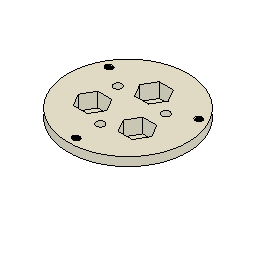
bottom platform (Autodesk Fusion 360 design; units mm, degrees)
Autodesk Fusion 360 part; units mm, degrees
sketch "Sketch6" plane through (0, 0, 0) normal (0, 1, 0) x (1, 0, 0)
  circle A0 centre (0, 0) radius 32.5
  dimension "d28" = 65
  constraint coincident A0.centre origin
  measures "d28" diameter of A0
extrude "Extrude5" add sketch "Sketch6" along normal blind 10 makes body 1
sketch "Sketch7" plane through (0, 0, 0) normal (0, -1, 0) x (1, 0, 0)
  circle A0 centre (0, 0) radius 32.5
  circle A1 centre (0, 0) radius 6
  dimension "d31" = 12
  constraint coincident A0.centre A1.centre
  measures "d31" diameter of A1
extrude "Extrude6" add sketch "Sketch7" along normal blind 10 contours A1 bodies 1
fillet "Fillet5" radius 3 1 edges at (-5.594, 0, 2.1697) on bodies 1
sketch "Sketch8" plane through (0, -10, 0) normal (0, -1, 0) x (1, 0, 0)
  circle A0 centre (0, 0) radius 6
  circle A1 centre (0, 0) radius 3.175
  dimension "d36" = 6.35
  constraint coincident A0.centre A1.centre
  measures "d36" diameter of A1
extrude "Extrude7" cut sketch "Sketch8" against normal blind 15 contours A1 bodies 1
thread "Thread2" "ANSI Unified Screw Threads 0.25 1/4-20 UNC 3B" major diameter 6.35 minor diameter 5.1156 pitch 1.27 angle 60 modelled right hand crest width 0.3725 on face at (3.1592, 0, -0.3161) crest through (2.5578, -9.6825, 0) on bodies 1
sketch "Sketch9" plane through (0, 10, 0) normal (0, 1, 0) x (-1, 0, 0)
  circle A0 centre (0, 0) radius 32.5
  circle A1 centre (0, 0) radius 23
  circle A2 centre (0, 0) radius 15 construction
  line L0 (4.1095, -22.0963) -> (8.2024, -14.9927)
  line L1 (8.2024, -14.9927) -> (4.0969, -7.8964)
  line L2 (4.0969, -7.8964) -> (-4.1015, -7.9037)
  line L3 (-4.1015, -7.9037) -> (-8.1944, -15.0073)
  line L4 (-8.1944, -15.0073) -> (-4.0889, -22.1036)
  line L5 (-4.0889, -22.1036) -> (4.1095, -22.0963)
  line L6 (21.1868, 7.5108) -> (17.0812, 14.6071)
  line L7 (17.0812, 14.6071) -> (8.8829, 14.5998)
  line L8 (8.8829, 14.5998) -> (4.79, 7.4962)
  line L9 (4.79, 7.4962) -> (8.8955, 0.3998)
  line L10 (8.8955, 0.3998) -> (17.0939, 0.4071)
  line L11 (17.0939, 0.4071) -> (21.1868, 7.5108)
  line L12 (-17.0979, 14.5929) -> (-21.1907, 7.4892)
  line L13 (-21.1907, 7.4892) -> (-17.0852, 0.3929)
  line L14 (-17.0852, 0.3929) -> (-8.8869, 0.4002)
  line L15 (-8.8869, 0.4002) -> (-4.794, 7.5038)
  line L16 (-4.794, 7.5038) -> (-8.8995, 14.6002)
  line L17 (-8.8995, 14.6002) -> (-17.0979, 14.5929)
  point P0 (0.004, -15)
  dimension "d39" = 46
  dimension "d40" = 30
  dimension "d41" = 14.2
  dimension "d43" = 360
  constraint coincident A0.centre A1.centre
  constraint coincident A2 P0
  measures "d39" diameter of A1
  measures "d40" diameter of A2
  measures "d41" distance of L2 L5
extrude "Extrude8" cut sketch "Sketch9" against normal blind 8.382 contours L0 L1 L2 L3 L4 L5 | L6 L7 L8 L9 L10 L11 | L12 L13 L14 L15 L16 L17 bodies 1
sketch "Sketch11" plane through (0, 0, 0) normal (0, -1, 0) x (1, 0, 0)
  circle A0 centre (0, 0) radius 32.5
  circle A1 centre (0, 0) radius 9
  circle A2 centre (0, 0) radius 27.5
  dimension "d65" = 55
  constraint concentric A0 A2
  measures "d65" diameter of A2
extrude "Extrude9" cut sketch "Sketch11" against normal blind 5 contours A0 bodies 1
sketch "Sketch12" plane through (0, 5, 0) normal (0, -1, 0) x (1, 0, 0)
  circle A0 centre (0, 0) radius 27.5
  circle A1 centre (0, 0) radius 32.5
  circle A2 centre (25.9808, -15) radius 2
  circle A3 centre (0, 30) radius 2
  line L0 (-28.1458, 16.25) -> (0, 0) construction
  line L1 (0, 0) -> (28.1458, -16.25) construction
  line L2 (0, 0) -> (0, 32.5) construction
  line L3 (23.8157, -13.75) -> (28.1458, -16.25) construction
  line L4 (0, 27.5) -> (0, 32.5) construction
  circle A4 centre (-25.9808, -15) radius 2
  dimension "d68" = 4
  dimension "d69" = 4
  dimension "d78" = 60
  constraint coincident A1 L0.start
  constraint coincident A0.centre A1.centre
  constraint coincident A1 L1.end
  constraint parallel L0 L1
  constraint coincident A1 L2.end
  constraint vertical L2
  constraint coincident A0 L3.start
  constraint coincident L1 L3.start
  constraint midpoint A2.centre L3
  constraint coincident L2 L4.start
  constraint coincident A0 L4.start
  constraint midpoint A3.centre L4
  constraint symmetric A2 L2 A4
  measures "d68" diameter of A2
  measures "d69" diameter of A3
  measures "d78" angle of L0 L2
extrude "Extrude10" cut sketch "Sketch12" against normal blind 5 contours A2 | A3 | A4 bodies 1
thread "Thread4" "ANSI Unified Screw Threads 0.164(#8) 8-32 UNC 3B" major diameter 4.1656 minor diameter 3.4163 pitch 0.7937 angle 60 modelled right hand crest width 0.2414 on face at (27.9783, 8.3333, -15.0997) crest through (27.6889, 5.1984, -15) on face at (-23.9832, 8.3333, -15.0997) crest through (-24.2726, 5.1984, -15) on face at (1.9975, 8.3333, 29.9003) crest through (1.7082, 5.1984, 30) on bodies 1
sketch "Sketch13" plane through (0, 0, 0) normal (0, -1, 0) x (1, 0, 0)
  circle A0 centre (0, 0) radius 27.5
  circle A1 centre (0, 0) radius 9
  line L0 (-8.2024, -14.9927) -> (-4.1095, -22.0963)
  line L1 (-4.1095, -22.0963) -> (4.0889, -22.1036)
  line L2 (4.0889, -22.1036) -> (8.1944, -15.0073)
  line L3 (8.1944, -15.0073) -> (4.1015, -7.9037)
  line L4 (4.1015, -7.9037) -> (-4.0969, -7.8964)
  line L5 (-4.0969, -7.8964) -> (-8.2024, -14.9927)
  line L6 (-17.0812, 14.6071) -> (-21.1868, 7.5108)
  line L7 (-21.1868, 7.5108) -> (-17.0939, 0.4071)
  line L8 (-17.0939, 0.4071) -> (-8.8955, 0.3998)
  line L9 (-8.8955, 0.3998) -> (-4.79, 7.4962)
  line L10 (-4.79, 7.4962) -> (-8.8829, 14.5998)
  line L11 (-8.8829, 14.5998) -> (-17.0812, 14.6071)
  line L12 (21.1907, 7.4892) -> (17.0979, 14.5929)
  line L13 (17.0979, 14.5929) -> (8.8995, 14.6002)
  line L14 (8.8995, 14.6002) -> (4.794, 7.5038)
  line L15 (4.794, 7.5038) -> (8.8869, 0.4002)
  line L16 (8.8869, 0.4002) -> (17.0852, 0.3929)
  line L17 (17.0852, 0.3929) -> (21.1907, 7.4892)
  circle A2 centre (0, 0) radius 32.5
  line L18 (0, 32.5) -> (0, -32.5) construction
  line L19 (-17.1424, 21.5032) -> (0, 9.5)
  line L20 (17.1424, 21.5032) -> (0, 9.5)
  line L21 (-10.0511, -25.5974) -> (-8.2272, -4.75)
  line L22 (-27.1935, 4.0941) -> (-8.2272, -4.75)
  line L23 (27.1935, 4.0941) -> (8.2272, -4.75)
  line L24 (10.0511, -25.5974) -> (8.2272, -4.75)
  spline S0 degree 3 poles (23.9261, -15.3413) (23.9965, -15.5962) (24.115, -15.8353) (24.432, -16.2447) (24.624, -16.4135) (25.0536, -16.6608) (25.2849, -16.7405) (25.6924, -16.7949) (25.862, -16.7938) (26.1902, -16.7441) (26.3473, -16.6973) (26.4954, -16.6288) knots 0 0 0 0 0.079347 0.079347 0.155456 0.155456 0.228326 0.228326 0.279114 0.279114 0.328226 0.328226 0.328226 0.328226
  arc A3 (26.4954, -16.6288) -> (27.3444, -13.9712) centre (25.9808, -15) ccw
  spline S1 degree 3 poles (27.3444, -13.9712) (27.2323, -13.7751) (27.0822, -13.6032) (26.7172, -13.3183) (26.5032, -13.2113) (26.0362, -13.0802) (25.7865, -13.0615) (25.3537, -13.1118) (25.1715, -13.1602) (24.8207, -13.3083) (24.6544, -13.4087) (24.5045, -13.5307) knots 0 0 0 0 0.06777 0.06777 0.138771 0.138771 0.213001 0.213001 0.26909 0.26909 0.326867 0.326867 0.326867 0.326867
  spline S2 degree 3 poles (-2.0546, 29.6587) (-1.9843, 29.4038) (-1.8658, 29.1647) (-1.5488, 28.7553) (-1.3567, 28.5865) (-0.9271, 28.3392) (-0.6958, 28.2595) (-0.2884, 28.2051) (-0.1188, 28.2062) (0.2094, 28.2559) (0.3666, 28.3027) (0.5146, 28.3712) knots 0 0 0 0 0.079347 0.079347 0.155456 0.155456 0.228326 0.228326 0.279114 0.279114 0.328226 0.328226 0.328226 0.328226
  arc A4 (0.5146, 28.3712) -> (1.3636, 31.0288) centre (0, 30) ccw
  spline S3 degree 3 poles (1.3636, 31.0288) (1.2516, 31.2249) (1.1015, 31.3968) (0.7364, 31.6817) (0.5225, 31.7887) (0.0554, 31.9198) (-0.1943, 31.9385) (-0.627, 31.8882) (-0.8092, 31.8398) (-1.1601, 31.6917) (-1.3263, 31.5913) (-1.4763, 31.4693) knots 0 0 0 0 0.06777 0.06777 0.138771 0.138771 0.213001 0.213001 0.26909 0.26909 0.326867 0.326867 0.326867 0.326867
  spline S4 degree 3 poles (-28.0354, -15.3413) (-27.965, -15.5962) (-27.8465, -15.8353) (-27.5296, -16.2447) (-27.3375, -16.4135) (-26.9079, -16.6608) (-26.6766, -16.7405) (-26.2692, -16.7949) (-26.0995, -16.7938) (-25.7713, -16.7441) (-25.6142, -16.6973) (-25.4661, -16.6288) knots 0 0 0 0 0.079347 0.079347 0.155456 0.155456 0.228326 0.228326 0.279114 0.279114 0.328226 0.328226 0.328226 0.328226
  arc A5 (-25.4661, -16.6288) -> (-24.6172, -13.9712) centre (-25.9808, -15) ccw
  spline S5 degree 3 poles (-24.6172, -13.9712) (-24.7292, -13.7751) (-24.8793, -13.6032) (-25.2443, -13.3183) (-25.4583, -13.2113) (-25.9253, -13.0802) (-26.175, -13.0615) (-26.6078, -13.1118) (-26.79, -13.1602) (-27.1408, -13.3083) (-27.3071, -13.4087) (-27.457, -13.5307) knots 0 0 0 0 0.06777 0.06777 0.138771 0.138771 0.213001 0.213001 0.26909 0.26909 0.326867 0.326867 0.326867 0.326867
  arc A6 (-27.457, -13.5307) -> (-28.0354, -15.3413) centre (-25.9808, -15) ccw
  arc A7 (-1.4763, 31.4693) -> (-2.0546, 29.6587) centre (0, 30) ccw
  arc A8 (24.5045, -13.5307) -> (23.9261, -15.3413) centre (25.9808, -15) ccw
  dimension "d72" = 55
  dimension "d73" = 23
  dimension "d75" = 360
  constraint coincident A2 L18.start
  constraint coincident A2 L18.end
  constraint vertical L18
  constraint coincident A0 L19.start
  constraint coincident L18 L19.end
  constraint symmetric L18 L19.start L20.start
  constraint symmetric L18 L19.end L20.end
  measures "d72" angle of L18 L19
  measures "d73" distance of L18.start L19.end
extrude "Extrude11" cut sketch "Sketch13" against normal blind 5 contours A0 L23 L24 | A0 L19 L20 | A0 L21 L22 bodies 1
sketch "Sketch10" plane through (0, 1.618, 0) normal (0, 1, 0) x (-1, 0, 0)
  line L0 (-8.8995, 14.6002) -> (-17.0979, 14.5929)
  line L1 (-17.0979, 14.5929) -> (-21.1907, 7.4892)
  line L2 (-21.1907, 7.4892) -> (-17.0852, 0.3929)
  line L3 (-17.0852, 0.3929) -> (-8.8869, 0.4002)
  line L4 (-8.8869, 0.4002) -> (-4.794, 7.5038)
  line L5 (-4.794, 7.5038) -> (-8.8995, 14.6002)
  line L6 (-4.0889, -22.1036) -> (4.1095, -22.0963)
  line L7 (4.1095, -22.0963) -> (8.2024, -14.9927)
  line L8 (8.2024, -14.9927) -> (4.0969, -7.8964)
  line L9 (4.0969, -7.8964) -> (-4.1015, -7.9037)
  line L10 (-4.1015, -7.9037) -> (-8.1944, -15.0073)
  line L11 (-8.1944, -15.0073) -> (-4.0889, -22.1036)
  line L12 (17.0939, 0.4071) -> (21.1868, 7.5108)
  line L13 (21.1868, 7.5108) -> (17.0812, 14.6071)
  line L14 (17.0812, 14.6071) -> (8.8829, 14.5998)
  line L15 (8.8829, 14.5998) -> (4.79, 7.4962)
  line L16 (4.79, 7.4962) -> (8.8955, 0.3998)
  line L17 (8.8955, 0.3998) -> (17.0939, 0.4071)
  line L18 (17.0939, 0.4071) -> (21.1868, 7.5108)
  line L19 (21.1868, 7.5108) -> (17.0812, 14.6071)
  line L20 (17.0812, 14.6071) -> (8.8829, 14.5998)
  line L21 (8.8829, 14.5998) -> (4.79, 7.4962)
  line L22 (4.79, 7.4962) -> (8.8955, 0.3998)
  line L23 (8.8955, 0.3998) -> (17.0939, 0.4071)
  line L24 (4.1095, -22.0963) -> (8.2024, -14.9927)
  line L25 (8.2024, -14.9927) -> (4.0969, -7.8964)
  line L26 (4.0969, -7.8964) -> (-4.1015, -7.9037)
  line L27 (-4.1015, -7.9037) -> (-8.1944, -15.0073)
  line L28 (-8.1944, -15.0073) -> (-4.0889, -22.1036)
  line L29 (-4.0889, -22.1036) -> (4.1095, -22.0963)
  line L30 (-8.8869, 0.4002) -> (-4.794, 7.5038)
  line L31 (-4.794, 7.5038) -> (-8.8995, 14.6002)
  line L32 (-8.8995, 14.6002) -> (-17.0979, 14.5929)
  line L33 (-17.0979, 14.5929) -> (-21.1907, 7.4892)
  line L34 (-21.1907, 7.4892) -> (-17.0852, 0.3929)
  line L35 (-17.0852, 0.3929) -> (-8.8869, 0.4002)
  circle A0 centre (12.9884, 7.5035) radius 3.5
  circle A1 centre (0.004, -15) radius 3.5
  circle A2 centre (-12.9924, 7.4965) radius 3.5
  point P0 (12.9884, 7.5035)
  point P1 (0.004, -15)
  point P2 (-12.9924, 7.4965)
  dimension "d50" = 7
  dimension "d51" = 7
  dimension "d52" = 7
  constraint coincident L16.end L17.start
  constraint coincident L12.start L17.end
  constraint coincident L6.start L11.end
  constraint coincident L6.end L7.start
  constraint coincident L3.end L4.start
  constraint coincident L2.end L3.start
  constraint coincident P0 A0.centre
  constraint coincident P1 A1.centre
  constraint coincident P2 A2.centre
  measures "d50" diameter of A0
  measures "d51" diameter of A1
  measures "d52" diameter of A2
fillet "Fillet7" radius 2 9 edges at (-17.1424, 2.5, 21.5032) (-27.1935, 2.5, 4.0941) (0, 2.5, 9.5) (17.1424, 2.5, 21.5032) (27.1935, 2.5, 4.0941) (8.2272, 2.5, -4.75) (10.0511, 2.5, -25.5974) (-10.0511, 2.5, -25.5974) (-8.2272, 2.5, -4.75) on bodies 1
sketch "Sketch14" plane through (0, 10, 0) normal (0, 1, 0) x (-1, 0, 0)
  line L0 (8.2024, -14.9927) -> (4.1095, -22.0963)
  line L1 (4.1095, -22.0963) -> (-4.0889, -22.1036)
  line L2 (-4.0889, -22.1036) -> (-8.1944, -15.0073)
  line L3 (-8.1944, -15.0073) -> (-4.1015, -7.9037)
  line L4 (-4.1015, -7.9037) -> (4.0969, -7.8964)
  line L5 (4.0969, -7.8964) -> (8.2024, -14.9927)
  line L6 (17.0812, 14.6071) -> (21.1868, 7.5108)
  line L7 (21.1868, 7.5108) -> (17.0939, 0.4071)
  line L8 (17.0939, 0.4071) -> (8.8955, 0.3998)
  line L9 (8.8955, 0.3998) -> (4.79, 7.4962)
  line L10 (4.79, 7.4962) -> (8.8829, 14.5998)
  line L11 (8.8829, 14.5998) -> (17.0812, 14.6071)
  line L12 (-21.1907, 7.4892) -> (-17.0979, 14.5929)
  line L13 (-17.0979, 14.5929) -> (-8.8995, 14.6002)
  line L14 (-8.8995, 14.6002) -> (-4.794, 7.5038)
  line L15 (-4.794, 7.5038) -> (-8.8869, 0.4002)
  line L16 (-8.8869, 0.4002) -> (-17.0852, 0.3929)
  line L17 (-17.0852, 0.3929) -> (-21.1907, 7.4892)
  circle A0 centre (0, 0) radius 32.5
  circle A1 centre (0, 0) radius 25
  circle A2 centre (0.004, -15) radius 3.5
  circle A3 centre (12.9884, 7.5035) radius 3.5
  circle A4 centre (-12.9924, 7.4965) radius 3.5
  circle A5 centre (0.004, -15) radius 4.9784
  circle A6 centre (-12.9924, 7.4965) radius 4.9784
  circle A7 centre (12.9884, 7.5035) radius 4.9784
  line L18 (0, 0) -> (-0.0223, 25) construction
  line L19 (0, 0) -> (21.6618, -12.4807) construction
  line L20 (0, 0) -> (-21.6395, -12.5193) construction
  circle A8 centre (13.8635, -7.9877) radius 2.3
  circle A9 centre (-0.0142, 16) radius 2.3
  circle A10 centre (-13.8493, -8.0123) radius 2.3
  spline S0 degree 3 poles (-23.9261, -15.3413) (-23.9965, -15.5962) (-24.115, -15.8353) (-24.432, -16.2447) (-24.624, -16.4135) (-25.0536, -16.6608) (-25.2849, -16.7405) (-25.6924, -16.7949) (-25.862, -16.7938) (-26.1902, -16.7441) (-26.3473, -16.6973) (-26.4954, -16.6288) knots 0 0 0 0 0.079347 0.079347 0.155456 0.155456 0.228326 0.228326 0.279114 0.279114 0.328226 0.328226 0.328226 0.328226
  arc A11 (-27.3444, -13.9712) -> (-26.4954, -16.6288) centre (-25.9808, -15) ccw
  spline S1 degree 3 poles (-27.3444, -13.9712) (-27.2323, -13.7751) (-27.0822, -13.6032) (-26.7172, -13.3183) (-26.5032, -13.2113) (-26.0362, -13.0802) (-25.7865, -13.0615) (-25.3537, -13.1118) (-25.1715, -13.1602) (-24.8207, -13.3083) (-24.6544, -13.4087) (-24.5045, -13.5307) knots 0 0 0 0 0.06777 0.06777 0.138771 0.138771 0.213001 0.213001 0.26909 0.26909 0.326867 0.326867 0.326867 0.326867
  spline S2 degree 3 poles (2.0546, 29.6587) (1.9843, 29.4038) (1.8658, 29.1647) (1.5488, 28.7553) (1.3567, 28.5865) (0.9271, 28.3392) (0.6958, 28.2595) (0.2884, 28.2051) (0.1188, 28.2062) (-0.2094, 28.2559) (-0.3666, 28.3027) (-0.5146, 28.3712) knots 0 0 0 0 0.079347 0.079347 0.155456 0.155456 0.228326 0.228326 0.279114 0.279114 0.328226 0.328226 0.328226 0.328226
  arc A12 (-1.3636, 31.0288) -> (-0.5146, 28.3712) centre (0, 30) ccw
  spline S3 degree 3 poles (-1.3636, 31.0288) (-1.2516, 31.2249) (-1.1015, 31.3968) (-0.7364, 31.6817) (-0.5225, 31.7887) (-0.0554, 31.9198) (0.1943, 31.9385) (0.627, 31.8882) (0.8092, 31.8398) (1.1601, 31.6917) (1.3263, 31.5913) (1.4763, 31.4693) knots 0 0 0 0 0.06777 0.06777 0.138771 0.138771 0.213001 0.213001 0.26909 0.26909 0.326867 0.326867 0.326867 0.326867
  spline S4 degree 3 poles (28.0354, -15.3413) (27.965, -15.5962) (27.8465, -15.8353) (27.5296, -16.2447) (27.3375, -16.4135) (26.9079, -16.6608) (26.6766, -16.7405) (26.2692, -16.7949) (26.0995, -16.7938) (25.7713, -16.7441) (25.6142, -16.6973) (25.4661, -16.6288) knots 0 0 0 0 0.079347 0.079347 0.155456 0.155456 0.228326 0.228326 0.279114 0.279114 0.328226 0.328226 0.328226 0.328226
  arc A13 (24.6172, -13.9712) -> (25.4661, -16.6288) centre (25.9808, -15) ccw
  spline S5 degree 3 poles (24.6172, -13.9712) (24.7292, -13.7751) (24.8793, -13.6032) (25.2443, -13.3183) (25.4583, -13.2113) (25.9253, -13.0802) (26.175, -13.0615) (26.6078, -13.1118) (26.79, -13.1602) (27.1408, -13.3083) (27.3071, -13.4087) (27.457, -13.5307) knots 0 0 0 0 0.06777 0.06777 0.138771 0.138771 0.213001 0.213001 0.26909 0.26909 0.326867 0.326867 0.326867 0.326867
  arc A14 (28.0354, -15.3413) -> (27.457, -13.5307) centre (25.9808, -15) ccw
  arc A15 (2.0546, 29.6587) -> (1.4763, 31.4693) centre (0, 30) ccw
  arc A16 (-23.9261, -15.3413) -> (-24.5045, -13.5307) centre (-25.9808, -15) ccw
  dimension "d81" = 50
  dimension "d82" = 9.9568
  dimension "d83" = 9.9568
  dimension "d84" = 9.9568
  dimension "d86" = 120
  dimension "d87" = 120
  dimension "d88" = 4.6
  dimension "d89" = 9
  dimension "d91" = 360
  constraint coincident A0.centre A1.centre
  constraint concentric A2 A5
  constraint concentric A4 A6
  constraint concentric A3 A7
  constraint coincident A1 L18.end
  constraint perpendicular L16 L18
  constraint coincident A1 L20.end
  constraint coincident L19 A8.centre
  measures "d81" diameter of A1
  measures "d82" diameter of A5
  measures "d83" diameter of A6
  measures "d84" diameter of A7
  measures "d86" angle of L19 L20
  measures "d87" angle of L18 L19
  measures "d88" diameter of A8
  measures "d89" distance of L19.end A8.centre
extrude "Extrude13" add sketch "Sketch14" along normal blind 2.794 separate body contours L0 L1 L2 L3 L4 L5 | L6 L7 L8 L9 L10 L11 | L12 L13 L14 L15 L16 L17 | A1 makes body 2
extrude "Extrude12" cut sketch "Sketch14" against normal blind 5 contours A8 | A9 | A10 bodies 1
move_face "OffsetFaces1" offset 2 1 faces at (-32.3385, 8.3333, -3.236) on bodies 1
hidden bodies 2
